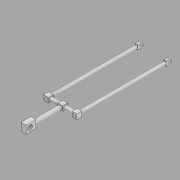
# Autodesk Inventor part: connectingRod2
Saved by Autodesk Inventor 2020 (Build 240168000, 168)
## iProperties
Company: Dibujo Computarizado AD2019
Created: 2019-11-16
Part Number: connectingRod2
Material: Genérico
Document SubType Name: Modeling
Designer: Gerardo Naranjo
Density: 1 g/cm^3
Appearance: Valor por defecto
Author: Gerardo Naranjo
Autodesk Inventor part; units mm, degrees
ref_plane "XZ Plane" through (0, 0, 0) normal (0, 1, 0) x (-1, 0, 0)
sketch "Boceto1" plane through (0, 0, 0) normal (0, 0, 1) x (1, 0, 0)
  line L0 (-2.3813, -2.3813) -> (2.3813, -2.3813)
  line L1 (2.3813, -2.3813) -> (2.3813, 2.3813)
  line L2 (2.3813, 2.3813) -> (-2.3813, 2.3813)
  line L3 (-2.3813, 2.3813) -> (-2.3813, -2.3813)
  line L4 (-2.3813, -2.3813) -> (2.3813, 2.3813) construction
  line L5 (2.3813, -2.3813) -> (-2.3813, 2.3813) construction
  circle A0 centre (0, 0) radius 1.5875
  dimension "d0" = 4.7625
  dimension "d1" = 4.7625
  dimension "d2" = 3.175
  constraints: 12 end point, 2 midpoint, 2 parallel, 1 centre point, 1 coincident, 1 horizontal, 1 perpendicular
  measures "d0" distance of L2.end L1.end
  measures "d1" distance of L1.end L0.end
  measures "d2" diameter of A0
extrude "Extrusión1" add sketch "Boceto1" along normal mid plane 4.7625
sketch "Boceto2" plane through (2.3813, -2.3813, 2.3813) normal (1, 0, 0) x (0, 0, -1)
  circle A0 centre (2.3813, 2.3813) radius 1.5875
  dimension "d5" = 3.175
  constraints: 1 centre point, 1 coincident
  measures "d5" diameter of A0
extrude "Extrusión2" add sketch "Boceto2" along normal blind 9.1281
sketch "Boceto3" plane through (-2.3813, -2.3813, 2.3813) normal (-1, 0, 0) x (0, 0, 1)
  circle A0 centre (-2.3813, 2.3813) radius 1.5875
  dimension "d8" = 3.175
  constraints: 1 centre point, 1 coincident
  measures "d8" diameter of A0
extrude "Extrusión3" add sketch "Boceto3" along normal blind 9.1281
sketch "Boceto4" plane through (0, 0, 0) normal (0, 0, 1) x (1, 0, 0)
  line L0 (-16.2719, -2.3812) -> (-11.5094, -2.3812)
  line L1 (-11.5094, -2.3812) -> (-11.5094, 2.3813)
  line L2 (-11.5094, 2.3813) -> (-16.2719, 2.3813)
  line L3 (-16.2719, 2.3813) -> (-16.2719, -2.3812)
  line L4 (-16.2719, -2.3812) -> (-11.5094, 2.3813) construction
  line L5 (-11.5094, -2.3812) -> (-16.2719, 2.3813) construction
  line L6 (11.5094, -2.3812) -> (16.2719, -2.3812)
  line L7 (16.2719, -2.3812) -> (16.2719, 2.3813)
  line L8 (16.2719, 2.3813) -> (11.5094, 2.3813)
  line L9 (11.5094, 2.3813) -> (11.5094, -2.3812)
  line L10 (11.5094, -2.3812) -> (16.2719, 2.3813) construction
  line L11 (16.2719, -2.3812) -> (11.5094, 2.3813) construction
  circle A0 centre (-13.8906, 0) radius 1.1906
  circle A1 centre (13.8906, 0) radius 1.1906
  point P0 (0, 0)
  dimension "d11" = 4.7625
  dimension "d12" = 4.7625
  dimension "d13" = 4.7625
  dimension "d14" = 4.7625
  dimension "d15" = 13.8906
  dimension "d16" = 13.8906
  dimension "d17" = 2.3813
  dimension "d18" = 2.3813
  constraints: 24 end point, 4 midpoint, 4 parallel, 2 centre point, 2 coincident, 2 horizontal, 2 perpendicular
  measures "d11" distance of L2.end L1.end
  measures "d12" distance of L1.end L0.end
  measures "d13" distance of L8.end L7.end
  measures "d14" distance of L7.end L6.end
  measures "d15" distance of point (13.891, 0) point (0, 0)
  measures "d16" distance of point (0, 0) point (-13.891, 0)
  measures "d17" diameter of A0
  measures "d18" diameter of A1
extrude "Extrusión4" add sketch "Boceto4" along normal mid plane 4.7625
sketch "Boceto5" plane through (0, 0, 2.3813) normal (0, 0, 1) x (1, 0, 0)
  circle A0 centre (0, 0) radius 1.5875
  constraints: 1 centre point, 1 coincident
extrude "Extrusión5" add sketch "Boceto5" along normal blind 26.1938
sketch "Boceto6" plane through (0, 0, 0) normal (1, 0, 0) x (0, 1, 0)
  line L0 (-3.9687, 28.575) -> (3.9687, 28.575)
  line L1 (3.9687, 28.575) -> (3.9687, 38.1)
  line L2 (3.9687, 38.1) -> (-3.9688, 38.1)
  line L3 (-3.9688, 38.1) -> (-3.9687, 28.575)
  line L4 (-3.9687, 28.575) -> (3.9687, 38.1) construction
  line L5 (3.9687, 28.575) -> (-3.9688, 38.1) construction
  line L6 (2.3812, 2.3813) -> (-2.3812, 2.3813) projected
  circle A0 centre (0, 34.1313) radius 2.3812
  point P0 (0, 0)
  point P1 (0, 33.3375)
  dimension "d23" = 7.9375
  dimension "d24" = 9.525
  dimension "d25" = 30.9563
  dimension "d26" = 4.7625
  dimension "d27" = 3.9688
  constraints: 12 end point, 2 midpoint, 2 parallel, 1 centre point, 1 horizontal, 1 perpendicular
  measures "d23" distance of L2.end L1.end
  measures "d24" distance of L1.end L0.end
  measures "d25" distance from line of point (0, 33.338) L6
  measures "d26" diameter of A0
  measures "d27" distance from line of L2 A0.centre
extrude "Extrusión6" add sketch "Boceto6" along normal mid plane 4.7625
sketch "Boceto7" plane through (0, 0, -2.3813) normal (0, 0, -1) x (-1, 0, 0)
  circle A0 centre (13.8906, 0) radius 1.1906 construction
  circle A1 centre (-13.8906, 0) radius 1.1906 construction
  circle A2 centre (-13.8906, 0) radius 1.1906
  circle A3 centre (13.8906, 0) radius 1.1906
  point P0 (0, 0)
  constraints: 2 centre point, 2 coincident, 2 concentric
extrude "Extrusión7" add sketch "Boceto7" along normal blind 83.3438
ref_plane "Plano de trabajo1" through (13.8906, 0, 0) normal (1, 0, 0) x (0, 1, 0)
sketch "Boceto8" plane through (13.8906, 0, 0) normal (1, 0, 0) x (0, 1, 0)
  arc A0 (-2.3813, -88.9) -> (2.3813, -88.9) centre (0, -88.9) ccw
  line L0 (2.3813, -88.9) -> (2.3813, -85.725)
  line L1 (-2.3813, -88.9) -> (-2.3813, -85.725)
  line L2 (-1.1906, -85.725) -> (1.1906, -85.725) construction
  line L3 (2.3813, -85.725) -> (-2.3813, -85.725)
  circle A1 centre (0, -88.9) radius 1.1906
  point P0 (0, 0)
  dimension "d33" = 4.7625
  dimension "d34" = 88.9
  dimension "d35" = 2.3813
  constraints: 6 end point, 2 centre point, 2 point on circle, 2 tangent, 2 vertical, 1 coincident, 1 horizontal
  measures "d33" diameter of A0
  measures "d34" distance of A0.centre point (0, 0)
  measures "d35" diameter of A1
extrude "Extrusión8" add sketch "Boceto8" along normal mid plane 2.3813
ref_plane "Plano de trabajo2" through (-13.8906, 0, 0) normal (1, 0, 0) x (0, 1, 0)
sketch "Boceto9" plane through (-13.8906, 0, 0) normal (1, 0, 0) x (0, 1, 0)
  arc A0 (-2.3813, -88.9) -> (2.3813, -88.9) centre (0, -88.9) ccw construction
  line L0 (2.3813, -85.725) -> (2.3813, -88.9) construction
  line L1 (0, -85.725) -> (2.3813, -85.725) construction
  line L2 (-2.3813, -85.725) -> (0, -85.725) construction
  line L3 (0, -85.725) -> (2.3813, -85.725) construction
  line L4 (2.3813, -85.725) -> (2.3813, -88.9) construction
  arc A1 (-2.3813, -88.9) -> (2.3813, -88.9) centre (0, -88.9) ccw construction
  line L5 (-2.3813, -88.9) -> (-2.3813, -85.725) construction
  circle A2 centre (0, -88.9) radius 1.1906 construction
  arc A3 (-2.3813, -88.9) -> (2.3813, -88.9) centre (0, -88.9) ccw
  line L6 (2.3813, -88.9) -> (2.3813, -85.725) projected
  line L7 (2.3813, -88.9) -> (2.3813, -85.725)
  line L8 (2.3813, -85.725) -> (-2.3813, -85.725)
  line L9 (-2.3813, -85.725) -> (-2.3813, -88.9) projected
  line L10 (-2.3813, -85.725) -> (-2.3813, -88.9)
  circle A4 centre (0, -88.9) radius 1.1906
  point P0 (0, 0)
  constraints: 6 end point, 2 centre point, 2 coincident, 2 collinear, 2 point on circle, 1 concentric, 1 vertical
extrude "Extrusión9" add sketch "Boceto9" along normal mid plane 2.3813
equation "\"d16\" = d15"
